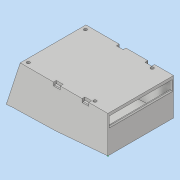
# Autodesk Inventor part: 仓库
Saved by Autodesk Inventor 2019 (Build 230136000, 136)
## iProperties
Created: 2020-11-07
Part Number: 仓库
Material: Generic
Document SubType Name: Modeling
Designer: Wang Hua
Density: 1 g/cm^3
Appearance: Default
Author: Wang Hua
Autodesk Inventor part; units mm, degrees
note: some values were not read from the file. Chosen so that the rebuilt part matches the saved one: direction of "孔1".
sketch "草图1" plane through (0, 0, 0) normal (0, 0, 1) x (1, 0, 0)
  line L0 (0, 0) -> (0, 3)
  line L1 (0, 0) -> (0, -6) construction
  line L2 (0, -6) -> (-106.5, -6) construction
  line L3 (-106.5, -6) -> (0, 3)
  line L4 (0, 0) -> (-54.9206, -4.6412)
  line L5 (-54.9206, -4.6412) -> (-106.5, -6)
  dimension "d0" = 3
  dimension "d1" = 6
  dimension "d2" = 106.5
  constraints: 12 end point, 2 vertical, 1 horizontal, 1 parallel
  measures "d0" distance of L0.start L0.end
  measures "d1" distance of L0.start L1.end
  measures "d2" distance of L1.end L2.end
extrude "拉伸1" add sketch "草图1" along normal blind 69
ref_plane "工作平面1" through (0, 38.6, 0) normal (0, 1, 0) x (-1, 0, 0)
sketch "草图2" plane through (0, 38.6, 0) normal (0, 1, 0) x (-1, 0, 0)
  line L0 (0, 0) -> (106.5, 0) construction
  line L1 (106.5, 0) -> (106.5, 69) construction
  line L2 (0, 69) -> (106.5, 69) construction
  line L3 (0, 0) -> (0, 69) construction
  line L4 (0, 0) -> (92, 0)
  line L5 (92, 0) -> (92, 1.5)
  line L6 (92, 1.5) -> (2, 1.5)
  line L7 (2, 1.5) -> (2, 67.5)
  line L8 (2, 67.5) -> (92, 67.5)
  line L9 (92, 67.5) -> (92, 69)
  line L10 (0, 0) -> (0, 69) projected
  line L11 (0, 69) -> (92, 69)
  line L12 (0, 69) -> (106.5, 69) projected
  line L13 (0, 0) -> (0, 69)
  dimension "d6" = 1.5
  dimension "d7" = 1.5
  dimension "d8" = 66
  dimension "d9" = 2
  dimension "d10" = 90
  constraints: 16 end point, 4 perpendicular, 4 point on line, 1 collinear, 1 vertical
  measures "d6" distance of L4.end L5.end
  measures "d7" distance of L8.end L9.end
  measures "d8" distance of L6.end L7.end
  measures "d9" distance between parallel lines of L3 L7
  measures "d10" distance between parallel lines of L7 L5
extrude "拉伸2" add sketch "草图2" against normal up to surface from surface at 0 surface through (0, 3, 0) normal (-0.0842069, 0.9964483, 0)
sketch "草图3" plane through (0, 38.6, 0) normal (0, 1, 0) x (-1, 0, 0)
  line L0 (2, 1.5) -> (92, 1.5) construction
  line L1 (2, 67.5) -> (2, 1.5) construction
  line L2 (92, 67.5) -> (2, 67.5) construction
  line L3 (92, 1.5) -> (2, 1.5)
  line L4 (2, 1.5) -> (2, 67.5)
  line L5 (92, 67.5) -> (2, 67.5)
  line L6 (92, 67.5) -> (92, 1.5)
  point P0 (0, 0)
  constraints: 8 end point, 3 collinear, 1 vertical
extrude "拉伸3" add sketch "草图3" against normal blind 3
sketch "草图4" plane through (-2, 2.831, 1.5) normal (-1, 0, 0) x (0, 0, 1)
  line L0 (66, 32.769) -> (0, 32.769) construction
  line L1 (0, 0) -> (0, 32.769) construction
  line L2 (66, 0) -> (0, 0) construction
  line L3 (66, 0) -> (66, 32.769) construction
  line L4 (66, -7.6056) -> (66, 32.769) projected
  line L5 (0, 32.769) -> (66, 32.769)
  line L6 (66, 32.769) -> (66, 22.769)
  line L7 (66, 22.769) -> (0, 22.769)
  line L8 (0, 22.769) -> (0, 32.769)
  point P0 (-1.5, -2.831)
  dimension "d15" = 10
  constraints: 8 end point, 2 parallel, 1 horizontal, 1 perpendicular, 1 point on line
  measures "d15" distance between parallel lines of L7 L0
extrude "拉伸4" cut sketch "草图4" against normal through all
sketch "草图5" plane through (0, 0, 69) normal (0, 0, 1) x (1, 0, 0)
  line L0 (-92, -4.7746) -> (-92, 38.6) construction
  line L1 (-92, -4.7746) -> (-106.5, -6) construction
  line L2 (-92, 38.6) -> (-92, -4.7746)
  line L3 (-106.5, -6) -> (-54.9206, -4.6412) projected
  line L4 (-92, -4.7746) -> (-92, 35.6) projected
  line L5 (-106.5, -6) -> (-92, -4.7746)
  line L6 (-92, -4.7746) -> (-92, 38.6) projected
  line L7 (-106.5, -6) -> (-92, 38.6)
  point P0 (0, 0)
  constraints: 6 end point, 1 collinear
extrude "拉伸5" add sketch "草图5" against normal blind 1.5
ref_plane "工作平面2" through (0, 0, 34.5) normal (0, 0, -1) x (-1, 0, 0)
mirror "镜像1" about plane through (0, 0, 34.5) normal (0, 0, -1) of "拉伸5"
sketch "草图7" plane through (0, 38.6, 69) normal (0, 1, 0) x (1, 0, 0)
  line L0 (-92, 69) -> (0, 69) projected
  line L1 (0, 69) -> (0, 0) construction
  line L2 (0, 34.5) -> (-92.7255, 34.5) construction
  line L3 (-92, 1.5) -> (-92, 67.5) projected
  point P0 (-18, 64.5)
  point P1 (-52, 64.5)
  point P2 (-88, 64.5)
  point P3 (-18, 4.5)
  point P4 (-52, 4.5)
  point P5 (-88, 4.5)
  point P6 (-92, 66.5)
  dimension "d22" = 4.5
  dimension "d23" = 4.5
  dimension "d24" = 4.5
  dimension "d25" = 34
  dimension "d26" = 36
  dimension "d27" = 60
  dimension "d35" = 4
  constraints: 3 symmetric about line, 2 end point, 1 horizontal, 1 midpoint
  measures "d22" distance from line of L0 point (-18, 64.5)
  measures "d23" distance from line of L0 point (-52, 64.5)
  measures "d24" distance from line of L0 point (-88, 64.5)
  measures "d25" distance of point (-52, 64.5) point (-18, 64.5)
  measures "d26" distance of point (-88, 64.5) point (-52, 64.5)
  measures "d27" distance of point (-18, 4.5) point (-18, 64.5)
  measures "d35" distance from line of L3 point (-88, 64.5)
hole "孔1" at (-88, 38.6, 64.5) at (-88, 38.6, 4.5) at (-18, 38.6, 4.5) at (-18, 38.6, 64.5) direction (0, -1, 0) diameter 3.2 depth 3
fillet "圆角1" radius 1 1 edges at (0, 25.6, 34.5)
sketch "草图9" plane through (0, 0, 69) normal (0, 0, 1) x (1, 0, 0)
  point P0 (0, 0)
sketch "草图10" plane through (0, 0, 69) normal (0, 0, 1) x (1, 0, 0)
  line L0 (-92, 38.6) -> (-106.5, -6) construction
  line L1 (-92, 35.6) -> (-92, 38.6) construction
  line L2 (-92, -4.7746) -> (-92, 35.6) construction
  line L3 (-92, -4.7746) -> (-106.5, -6) construction
  line L4 (-106.5, -6) -> (-54.9206, -4.6412) projected
  line L5 (-106.5, -6) -> (-106.5, -5)
  line L6 (-127.8168, 0) -> (21.4009, 0) projected
  line L7 (-106.5, -5) -> (-80.7103, -3.8206)
  line L8 (-2, 2.831) -> (-106.5, -6) projected
  line L9 (-106.5, -6) -> (-92, 38.6) projected
  line L10 (-106.5, -6) -> (-80.7103, -3.8206)
  line L11 (-106.5, -6) -> (-106.5, -6.5)
  line L12 (-106.5, -6.5) -> (-80.7103, -3.8206)
  line L13 (-106.5, -5.2) -> (-80.7103, -3.8206)
  point P0 (0, 0)
  dimension "d37" = 1
  dimension "d38" = 25.7897
  dimension "d42" = 0.5
  dimension "d55" = 0.2
  constraints: 12 end point, 2 point on line, 1 perpendicular, 1 vertical
  measures "d37" distance of L0.end L5.end
  measures "d38" horizontal distance of L5.end L7.end
  measures "d42" distance of L0.end L11.end
  measures "d55" distance of L13.start L5.end
extrude "拉伸7" add sketch "草图10" against normal up to surface (69 mm away) from surface at 0 contours L8 L12 L4 | L9 L13 L8 | L5 L13 L9 | L4 L12 L11 | L5 L7 L9 L13 | L13 L9 L7
sketch "草图11" plane through (-54.9206, -4.6412, 0) normal (0.0263351, -0.9996532, 0) x (0.9996532, 0.0263351, 0)
  point P0 (55.0238, 0)
ref_plane "工作平面3" through (0, -6, 0) normal (0, 1, 0) x (-1, 0, 0)
sketch "草图12" plane through (0, 38.6, 69) normal (0, 1, 0) x (1, 0, 0)
  line L0 (0, 0) -> (-92, 0) projected
  line L1 (-53.5, 0) -> (-53.5, 3)
  line L2 (-92, 1.5) -> (-92, 67.5) projected
  line L3 (-54.9206, 0) -> (0, 0) projected
  line L4 (-57, 3) -> (-50, 3)
  line L5 (-50, 3) -> (-50, 0)
  line L6 (-50, 0) -> (-57, 0)
  line L7 (-57, 0) -> (-57, 3)
  line L8 (-92, 1.5) -> (0, 1.5) projected
  line L9 (-57, 3) -> (-50, 0) construction
  line L10 (-50, 3) -> (-57, 0) construction
  line L11 (-20, 3) -> (-27, 3)
  line L12 (-27, 3) -> (-27, 0)
  line L13 (-27, 0) -> (-20, 0)
  line L14 (-20, 0) -> (-20, 3)
  line L15 (-20, 3) -> (-27, 0) construction
  line L16 (-27, 3) -> (-20, 0) construction
  point P0 (0, 69)
  point P1 (-53.5, 1.5)
  point P2 (-23.5, 1.5)
  dimension "d43" = 38.5
  dimension "d44" = 3
  dimension "d45" = 7
  dimension "d46" = 68.5
  dimension "d47" = 3
  dimension "d48" = 7
  constraints: 26 end point, 5 midpoint, 4 parallel, 4 point on line, 2 horizontal, 2 perpendicular, 1 vertical
  measures "d43" distance between parallel lines of L1 L2
  measures "d44" distance of L1.start L1.end
  measures "d45" distance of L4.start L4.end
  measures "d46" distance from line of L2 point (-23.5, 1.5)
  measures "d47" distance of L11.end L12.end
  measures "d48" distance of L11.start L11.end
extrude "拉伸8" cut sketch "草图12" against normal blind 3.5 contours L0 L12 L8 L14 | L8 L12 L11 L14 | L0 L1 L8 L5 | L0 L7 L8 L1 | L8 L1 L4 L5 | L8 L7 L4 L1
ref_plane "工作平面4" through (0, 0, 34.5) normal (0, 0, 1) x (1, 0, 0)
mirror "镜像2" about plane through (0, 0, 34.5) normal (0, 0, 1) of "拉伸8"
extrude "拉伸9" cut sketch "草图10" along normal up to surface (66 mm away) from surface at -67.5 contours L5 L7 L9 L13 | L13 L9 L7
